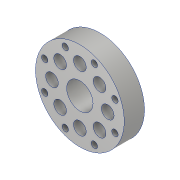
# Autodesk Inventor part: 조인트4베어링관절혼
Saved by Autodesk Inventor 2020.5 (Build 245400000, 400)
## iProperties
Created: 2021-07-15
Part Number: 조인트4베어링관절혼
Material: 알루미늄 6061
Document SubType Name: Modeling
Designer: user
Density: 2.7 g/cm^3
Appearance: 알루미늄 - 평지
Mass: 15.9074 g
Surface Area: 40.0195 cm^2
Volume: 5.89162 cm^3
Author: user
Autodesk Inventor part; units mm, degrees
ref_plane "YZ Plane" through (0, 0, 0) normal (1, 0, 0) x (0, 1, 0)
ref_plane "XZ Plane" through (0, 0, 0) normal (0, 1, 0) x (-1, 0, 0)
ref_plane "XY Plane" through (0, 0, 0) normal (0, 0, 1) x (1, 0, 0)
sketch "스케치3" plane through (0, 0, 0) normal (0, 0, 1) x (1, 0, 0)
  circle A0 centre (0, 0) radius 5.2
  circle A1 centre (0, 0) radius 17.5
  dimension "d13" = 10.4
  dimension "d14" = 35
  constraints: 2 centre point, 2 coincident
  measures "d13" diameter of A0
  measures "d14" diameter of A1
extrude "돌출3" add sketch "스케치3" along normal blind 8
sketch "스케치4" plane through (0, 0, 8) normal (0, 0, 1) x (1, 0, 0)
  circle A0 centre (0, 0) radius 11
  line L0 (0, 0) -> (0, 11)
  line L1 (0, 0) -> (11, 0) construction
  circle A1 centre (0, 11) radius 1.35
  circle A2 centre (-7.7782, 7.7782) radius 1.35
  circle A3 centre (-11, 0) radius 1.35
  circle A4 centre (-7.7782, -7.7782) radius 1.35
  circle A5 centre (0, -11) radius 1.35
  circle A6 centre (7.7782, -7.7782) radius 1.35
  circle A7 centre (11, 0) radius 1.35
  circle A8 centre (7.7782, 7.7782) radius 1.35
  dimension "d17" = 22
  dimension "d18" = 11
  dimension "d19" = 90
  dimension "d20" = 2.7
  dimension "d23" = 360
  constraints: 9 centre point, 4 end point, 2 coincident, 1 horizontal, 1 perpendicular, 1 vertical, 17 other
  measures "d17" diameter of A0
  measures "d18" distance of L0.start L0.end
  measures "d19" angle of L1 L0
  measures "d20" diameter of A1
extrude "돌출4" cut sketch "스케치4" against normal up to surface (8 mm away) contours A0 A7 | A0 A7 | A8 A0 | A0 A8 | A6 A0 | A0 A6 | A1 L0 A0 | A0 A1 | A5 A0 | A0 A5 | L0 A1 A0 | A4 A0 | A0 A4 | A2 A0 | A0 A2 | A3 A0 | A0 A3
sketch "스케치5" plane through (0, 0, 8) normal (0, 0, 1) x (1, 0, 0)
  circle A0 centre (7.7782, 7.7782) radius 1.35 projected
  circle A1 centre (11, 0) radius 1.35 projected
  circle A2 centre (0, -11) radius 1.35 projected
  circle A3 centre (-11, 0) radius 1.35 projected
  circle A4 centre (0, 11) radius 1.35 projected
  circle A5 centre (-7.7782, 7.7782) radius 1.35 projected
  circle A6 centre (-7.7782, -7.7782) radius 1.35 projected
  circle A7 centre (7.7782, -7.7782) radius 1.35 projected
  circle A8 centre (0, 0) radius 5.2 projected
  circle A9 centre (0, 0) radius 17.5 projected
  circle A10 centre (-11, 0) radius 2.5
  circle A11 centre (-7.7782, 7.7782) radius 2.5
  circle A12 centre (0, 11) radius 2.5
  circle A13 centre (7.7782, 7.7782) radius 2.5
  circle A14 centre (11, 0) radius 2.5
  circle A15 centre (7.7782, -7.7782) radius 2.5
  circle A16 centre (0, -11) radius 2.5
  circle A17 centre (-7.7782, -7.7782) radius 2.5
  dimension "d27" = 5
  dimension "d28" = 5
  dimension "d29" = 5
  dimension "d30" = 5
  dimension "d31" = 5
  dimension "d32" = 5
  dimension "d33" = 5
  dimension "d34" = 5
  constraints: 8 centre point, 8 coincident
  measures "d27" diameter of A10
  measures "d28" diameter of A11
  measures "d29" diameter of A12
  measures "d30" diameter of A13
  measures "d31" diameter of A14
  measures "d32" diameter of A15
  measures "d33" diameter of A16
  measures "d34" diameter of A17
extrude "돌출5" cut sketch "스케치5" against normal blind 4 contours A10 | A11 | A12 | A13 | A14 | A15 | A16 | A17
sketch "스케치6" plane through (0, 0, 8) normal (0, 0, 1) x (1, 0, 0)
  circle A0 centre (0, 0) radius 14
  line L0 (0, 0) -> (-5.7403, 13.8582)
  line L1 (0, 0) -> (15, 0) construction
  circle A1 centre (-5.7403, 13.8582) radius 1.25
  circle A2 centre (-13.8582, 5.7403) radius 1.25
  circle A3 centre (-13.8582, -5.7403) radius 1.25
  circle A4 centre (-5.7403, -13.8582) radius 1.25
  circle A5 centre (5.7403, -13.8582) radius 1.25
  circle A6 centre (13.8582, -5.7403) radius 1.25
  circle A7 centre (13.8582, 5.7403) radius 1.25
  circle A8 centre (5.7403, 13.8582) radius 1.25
  dimension "d37" = 28
  dimension "d38" = 15
  dimension "d39" = 112.5
  dimension "d40" = 2.5
  dimension "d43" = 360
  constraints: 9 centre point, 4 end point, 2 coincident, 1 equal length, 1 horizontal, 17 other
  measures "d37" diameter of A0
  measures "d38" distance of L0.start L0.end
  measures "d39" angle of L1 L0
  measures "d40" diameter of A1
extrude "돌출6" cut sketch "스케치6" against normal up to surface (8 mm away) contours A7 A0 | A0 A7 | A6 A0 | A0 A6 | A8 A0 | A0 A8 | A5 A0 | A0 A5 | A1 L0 A0 | A0 A1 | A4 A0 | A0 A4 | L0 A1 A0 | A3 A0 | A0 A3 | A2 A0 | A0 A2
